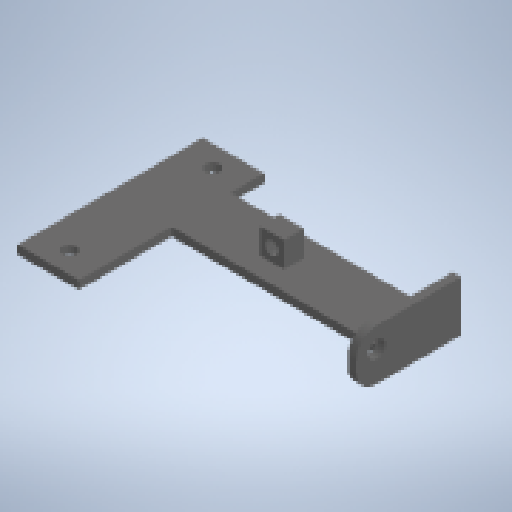
# Autodesk Inventor part: hand_motor_setter_cover_under
Saved by Autodesk Inventor 2024.1 (Build 281209000, 209)
## iProperties
Created: 2025-01-23
Part Number: hand_motor_setter_cover_under
Material: 一般
Document SubType Name: Modeling
Designer: hibik
Density: 1 g/cm^3
Appearance: 既定
Author: hibik
Autodesk Inventor part; units mm, degrees
ref_plane "YZ Plane" through (0, 0, 0) normal (1, 0, 0) x (0, 1, 0)
ref_plane "XZ Plane" through (0, 0, 0) normal (0, 1, 0) x (-1, 0, 0)
ref_plane "XY Plane" through (0, 0, 0) normal (0, 0, 1) x (1, 0, 0)
sketch "スケッチ1" plane through (0, 0, 0) normal (0, 1, 0) x (-1, 0, 0)
  line L0 (0, 0) -> (-14.7, 0)
  line L1 (-14.7, 0) -> (-14.7, -44.2)
  line L2 (-14.7, -44.2) -> (0, -44.2)
  line L3 (0, -44.2) -> (0, 0)
  line L4 (-14.7, -36.2) -> (-69.7, -36.2)
  line L5 (-69.7, -36.2) -> (-69.7, -22.1)
  line L6 (-69.7, -22.1) -> (-14.7, -22.1)
  line L7 (-14.7, -22.1) -> (-14.7, -36.2)
  line L8 (-7.35, -44.2) -> (-7.35, 0) construction
  circle A0 centre (-7.35, -39.2) radius 1.6
  circle A1 centre (-7.35, -5) radius 1.6
  point P0 (-14.7, -22.1)
  dimension "d0" = 14.7
  dimension "d1" = 44.2
  dimension "d2" = 22.1
  dimension "d3" = 14.1
  dimension "d4" = 3.2
  dimension "d5" = 3.2
  dimension "d6" = 5
  dimension "d7" = 5
  dimension "d20" = 55
  constraints: 18 end point, 4 parallel, 3 point on line, 2 centre point, 2 horizontal, 2 midpoint, 2 perpendicular
  measures "d0" distance of L2.end L1.end
  measures "d1" distance of L1.end L0.end
  measures "d2" distance between parallel lines of L2 L6
  measures "d3" distance between parallel lines of L6 L4
  measures "d4" diameter of A0
  measures "d5" diameter of A1
  measures "d6" distance of L8.start A0.centre
  measures "d7" distance from line of L0 A1.centre
  measures "d20" distance of L4.start L4.end
extrude "押し出し1" add sketch "スケッチ1" along normal blind 2
ref_plane "作業平面1" through (31, 0, -44.2) normal (-1, 0, 0) x (0, 0, 1)
sketch "スケッチ3" plane through (31, 0, -44.2) normal (-1, 0, 0) x (0, 0, 1)
  line L0 (22.1, 0) -> (8, 0) projected
  line L1 (8, 0) -> (8, 2) projected
  line L2 (22.1, 2) -> (8, 2) projected
  line L3 (22.1, 0) -> (22.1, 2) projected
  line L4 (17.45, 2) -> (12.65, 2)
  line L5 (12.65, 2) -> (12.65, 8)
  line L6 (12.65, 8) -> (17.45, 8)
  line L7 (17.45, 8) -> (17.45, 2)
  line L8 (22.1, 0) -> (8, 0) projected
  point P0 (44.2, 0)
  point P1 (15.05, 8)
  point P2 (15.05, 0)
  point P3 (12.65, 2)
  dimension "d11" = 4.8
  dimension "d12" = 6
  constraints: 8 end point, 2 midpoint, 2 parallel, 1 horizontal, 1 perpendicular, 1 point on line, 1 vertical alignment
  measures "d11" distance of L5.end L6.end
  measures "d12" distance of L6.end L4.start
extrude "押し出し2" add sketch "スケッチ3" against normal blind 5.9 contours L2 L5 L6 L7
sketch "スケッチ4" plane through (31, 2, -26.75) normal (0, 0, 1) x (1, 0, 0)
  circle A0 centre (2.9, 3) radius 1.6
  line L0 (5.9, 6) -> (5.9, 0) projected
  line L1 (0, 6) -> (5.9, 6) projected
  point P0 (-31, -2)
  dimension "d15" = 3.2
  dimension "d16" = 3
  dimension "d17" = 3
  constraints: 1 centre point
  measures "d15" diameter of A0
  measures "d16" distance from line of L0 A0.centre
  measures "d17" distance from line of L1 A0.centre
extrude "押し出し3" cut sketch "スケッチ4" against normal through all
sketch "スケッチ5" plane through (69.7, 0, -22.1) normal (1, 0, 0) x (0, 0, -1)
  circle A0 centre (-6, 7.1) radius 2 projected
  line L0 (0, 0) -> (14.1, 0) projected
  line L1 (14.1, 0) -> (14.1, 2) projected
  line L2 (0, 2) -> (14.1, 2) projected
  line L3 (0, 0) -> (0, 2) projected
  line L4 (14.1, 0) -> (22.1, 0) projected
  line L5 (14.1, 0) -> (-11, 0)
  line L6 (-11, 0) -> (-11, 12.1)
  line L7 (-11, 12.1) -> (14.1, 12.1)
  line L8 (14.1, 12.1) -> (14.1, 0)
  circle A1 centre (-6, 7.1) radius 5
  circle A2 centre (-6, 5) radius 5
  point P0 (-22.1, 0)
  point P1 (-11, 7.1)
  point P2 (-6, 12.1)
  point P3 (-11, 5)
  point P4 (-6, 0)
  dimension "d21" = 5
  dimension "d22" = 5
  constraints: 8 end point, 3 tangent, 2 centre point, 2 parallel, 1 coincident, 1 equal radius, 1 horizontal, 1 perpendicular
  measures "d21" distance from line of L6 A0.centre
  measures "d22" distance from line of L7 A0.centre
extrude "押し出し4" add sketch "スケッチ5" against normal blind 2 contours L3 L2 L1 L0 | L5 A2 A1 L7 L8 L2 L3 | A2 A1 | L6 A1 A2 | A1 A2 | A2 A1
fillet "フィレット1" radius 3 1 edges at (67.7, 2, -29.15)
equation "\"d22\" = d21"
